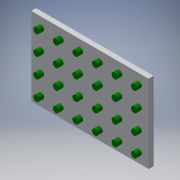
# Autodesk Inventor part: Rectangular
Saved by Autodesk Inventor 2018 (Build 220112000, 112)
## iProperties
Shininess: 64.0
Length Units: 11272
Angle Units: 11279
Time Units: 11290
Mass Units: 11286
Length Display Precision: 3
Angle Display Precision: 2
Compacted: True
Part Number: Rectangular
Document SubType Name: Modeling
Created: 2003-12-04
Designer: dischinger.b
Material: Generic
Density: 1 g/cm^3
Appearance: Cool White
Density: 0.0
Volumn: 0.0
Area: 0.0
PropertySet Name: Model Information
Control State: 0
Master: False
Checked Out: False
Author: dischinger.b
Autodesk Inventor part; units mm, degrees
ref_plane "YZ Plane" through (0, 0, 0) normal (1, 0, 0) x (0, 1, 0)
ref_plane "XZ Plane" through (0, 0, 0) normal (0, 1, 0) x (-1, 0, 0)
ref_plane "XY Plane" through (0, 0, 0) normal (0, 0, 1) x (1, 0, 0)
sketch "Sketch1" plane through (0, 0, 0) normal (0, 0, 1) x (1, 0, 0)
  line L0 (-38.3761, 21.7949) -> (114.0239, 21.7949)
  line L1 (114.0239, 21.7949) -> (114.0239, -79.8051)
  line L2 (114.0239, -79.8051) -> (-38.3761, -79.8051)
  line L3 (-38.3761, -79.8051) -> (-38.3761, 21.7949)
  dimension "d0" = 152.4
  dimension "d1" = 101.6
  constraints: 8 end point, 2 parallel, 1 horizontal, 1 perpendicular
  measures "d0" distance of L0.start L0.end
  measures "d1" distance of L2.end L0.start
extrude "Extrusion1" add sketch "Sketch1" along normal blind 6.35
sketch "Sketch2" plane through (0, 0, 6.35) normal (0, 0, 1) x (1, 0, 0)
  line L0 (-38.3761, -79.8051) -> (-38.3761, 21.7949) projected
  line L1 (114.0239, -79.8051) -> (-38.3761, -79.8051) projected
  circle A0 centre (-25.6761, -67.1051) radius 3.81
  dimension "d4" = 7.62
  dimension "d5" = 12.7
  dimension "d6" = 12.7
  constraints: 1 centre point
  measures "d4" diameter of A0
  measures "d5" distance from line of L1 A0.centre
  measures "d6" distance from line of L0 A0.centre
extrude "Extrusion2" add sketch "Sketch2" along normal blind 6.35
pattern_linear "Rectangular Pattern1" count 6 spacing 25.4 along (1, 0, 0) count 4 spacing 25.4 along (0, 1, 0) of "Extrusion2"
body "Solid1"
